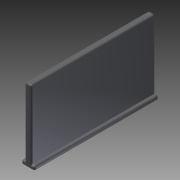
# Autodesk Inventor part: Medium Conveyor Belt Inserts
Saved by Autodesk Inventor 2013 (Build 170138000, 138)
## iProperties
Category: Motion
Company: Autodesk Inc.
Created: 2012-03-02
Part Number: Medium Conveyor Belt Inserts
Document SubType Name: Modeling
Designer: Autodesk Inc.
Density: 1.42 g/cm^3
Material: Acetal Resin, White
Catalog Web Link: http://www.vexrobotics.com/276-2214.html
Vendor: VEX
Mass: 2.52103 g
Surface Area: 20.2027 cm^2
Volume: 1.77538 cm^3
Author: Autodesk Inc.
Autodesk Inventor part; units mm, degrees
ref_plane "YZ Plane" through (0, 0, 0) normal (1, 0, 0) x (0, 1, 0)
ref_plane "XZ Plane" through (0, 0, 0) normal (0, 1, 0) x (-1, 0, 0)
ref_plane "XY Plane" through (0, 0, 0) normal (0, 0, 1) x (1, 0, 0)
sketch "Sketch1" plane through (0, 0, 0) normal (0, 0, 1) x (1, 0, 0)
  line L0 (3, 0.8) -> (3, -0.5)
  line L1 (3, -0.5) -> (-1, -0.5)
  line L2 (-1, -0.5) -> (-1, 0.8)
  line L3 (0, 0.8) -> (0, 21.8012)
  line L4 (0, 21.8012) -> (2, 21.8012)
  line L5 (2, 21.8012) -> (2, 0.8)
  line L6 (-1, 0.8) -> (0, 0.8)
  line L7 (2, 0.8) -> (3, 0.8)
  line L8 (-1, 0.8) -> (0, 0.8)
  line L9 (2, 0.8) -> (2.5, 0.8)
  point P0 (0, 0)
  point P1 (1, -0.5)
  point P2 (1, -0.5)
  dimension "d0" = 22.3012
  dimension "d1" = 4
  dimension "d2" = 1.3
  dimension "d3" = 1
  dimension "d4" = 1
  constraints: 20 end point, 2 midpoint, 1 other
  measures "d0" distance between parallel lines of L1 L4
  measures "d1" distance of L1.start L1.end
  measures "d2" distance from line of L9.end L1
  measures "d3" distance between parallel lines of L0 L5
  measures "d4" distance between parallel lines of L2 L3
extrude "Extrusion1" add sketch "Sketch1" along normal mid plane 37.9984
fillet "Fillet1" radius 0.508 22 edges at (2, 11.3006, 18.9992) (2, 21.8012, 0) (2, 11.3006, -18.9992) (2.5, 0.8, 18.9992) (-0.5, 0.8, 18.9992) (-1, 0.15, 18.9992) (1, -0.5, 18.9992) (3, 0.15, 18.9992) (3, 0.8, 0) (1, 21.8012, 18.9992) (0, 11.3006, 18.9992) (0, 21.8012, 0) (2.5, 0.8, -18.9992) (3, 0.15, -18.9992) (-0.5, 0.8, -18.9992) (-1, 0.15, -18.9992) (1, -0.5, -18.9992) (-1, 0.8, 0) (-1, -0.5, 0) (1, 21.8012, -18.9992) (3, -0.5, 0) (0, 11.3006, -18.9992)
equation "\"d4\" = d3"
body "Solid1"
